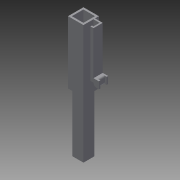
# Autodesk Inventor part: CraneArmLink1st
Saved by Autodesk Inventor 2015 (Build 190159000, 159)
## iProperties
Created: 2016-03-24
Part Number: CraneArmLink1st
Material: Generic
Document SubType Name: Modeling
Designer: Hatch
Density: 1 g/cm^3
Appearance: Default
Author: Hatch
Autodesk Inventor part; units mm, degrees
ref_plane "YZ Plane" through (0, 0, 0) normal (1, 0, 0) x (0, 1, 0)
ref_plane "XZ Plane" through (0, 0, 0) normal (0, 1, 0) x (-1, 0, 0)
ref_plane "XY Plane" through (0, 0, 0) normal (0, 0, 1) x (1, 0, 0)
sketch "Sketch1" plane through (0, 0, 0) normal (0, 1, 0) x (-1, 0, 0)
  line L0 (-7.125, 7.125) -> (7.125, 7.125)
  line L1 (7.125, 7.125) -> (7.125, -7.125)
  line L2 (7.125, -7.125) -> (-7.125, -7.125)
  line L3 (-7.125, -7.125) -> (-7.125, 7.125)
  line L4 (-7.125, 7.125) -> (7.125, -7.125) construction
  line L5 (7.125, 7.125) -> (-7.125, -7.125) construction
  point P0 (0, 0)
  dimension "d0" = 14.25
  dimension "d1" = 14.25
  constraints: 12 end point, 2 midpoint, 2 parallel, 1 horizontal, 1 perpendicular
  measures "d0" distance of L1.end L2.end
  measures "d1" distance of L0.end L1.end
extrude "Extrusion1" add sketch "Sketch1" along normal blind 76.2
sketch "Sketch2" plane through (0, 76.2, 0) normal (0, 1, 0) x (1, 0, 0)
  line L0 (10, -10) -> (-10, -10)
  line L1 (-10, -10) -> (-10, 10)
  line L2 (-10, 10) -> (10, 10)
  line L3 (10, 10) -> (10, -10)
  line L4 (10, -10) -> (-10, 10) construction
  line L5 (-10, -10) -> (10, 10) construction
  point P0 (0, 0)
  dimension "d4" = 20
  dimension "d5" = 20
  constraints: 12 end point, 2 midpoint, 2 parallel, 1 horizontal, 1 perpendicular
  measures "d4" distance of L1.end L2.end
  measures "d5" distance of L0.end L1.end
extrude "Extrusion2" add sketch "Sketch2" along normal blind 5
sketch "Sketch3" plane through (0, 81.2, 0) normal (0, 1, 0) x (1, 0, 0)
  line L0 (7.5, -7.5) -> (-7.5, -7.5)
  line L1 (-7.5, -7.5) -> (-7.5, 7.5)
  line L2 (-7.5, 7.5) -> (7.5, 7.5)
  line L3 (7.5, 7.5) -> (7.5, -7.5)
  line L4 (7.5, -7.5) -> (-7.5, 7.5) construction
  line L5 (-7.5, -7.5) -> (7.5, 7.5) construction
  line L6 (10, -10) -> (-10, -10)
  line L7 (-10, -10) -> (-10, 10)
  line L8 (-10, 10) -> (10, 10)
  line L9 (10, 10) -> (10, -10)
  line L10 (10, -10) -> (-10, 10) construction
  line L11 (-10, -10) -> (10, 10) construction
  point P0 (0, 0)
  dimension "d8" = 15
  dimension "d9" = 15
  constraints: 24 end point, 4 midpoint, 4 parallel, 2 horizontal, 2 perpendicular
  measures "d8" distance of L1.end L2.end
  measures "d9" distance of L0.end L1.end
extrude "Extrusion3" add sketch "Sketch3" along normal blind 76.2
sketch "Sketch4" plane through (10, 76.2, 10) normal (1, 0, 0) x (0, 0, -1)
  line L0 (20, 0) -> (20, 81.2) projected
  line L1 (15, 81.2) -> (15, 0)
  line L2 (0, 0) -> (20, 0) projected
  line L3 (15, 81.2) -> (13, 81.2)
  line L4 (17.5, 81.2) -> (2.5, 81.2) projected
  line L5 (13, 81.2) -> (13, 0)
  line L6 (13, 0) -> (15, 0)
  line L7 (20, 81.2) -> (0, 81.2) projected
  point P0 (10, -76.2)
  dimension "d12" = 2
  constraints: 8 end point, 3 point on line, 1 parallel, 1 perpendicular, 1 vertical
  measures "d12" distance of L1.start L3.end
extrude "Extrusion4" add sketch "Sketch4" along normal blind 10 contours L2 L5 L3 L1
sketch "Sketch5" plane through (10, 76.2, -3) normal (0, 0, 1) x (1, 0, 0)
  line L0 (0, 81.2) -> (10, 81.2) projected
  line L1 (10, 81.2) -> (8, 81.2)
  line L2 (8, 81.2) -> (8, 0)
  line L3 (8, 0) -> (10, 0)
  line L4 (10, 0) -> (10, 81.2)
  point P0 (-10, -76.2)
  dimension "d15" = 2
  constraints: 8 end point, 2 parallel, 1 perpendicular, 1 point on line
  measures "d15" distance of L0.end L1.end
extrude "Extrusion5" add sketch "Sketch5" along normal blind 8
sketch "Sketch6" plane through (20, 76.2, 10) normal (1, 0, 0) x (0, 0, -1)
  line L0 (5, 81.2) -> (3, 81.2)
  line L1 (3, 81.2) -> (3, 0)
  line L2 (3, 0) -> (5, 0)
  line L3 (5, 0) -> (5, 81.2)
  point P0 (10, -76.2)
  dimension "d18" = 2
  constraints: 8 end point, 2 parallel, 1 horizontal, 1 perpendicular
  measures "d18" distance of L0.start L0.end
extrude "Extrusion6" add sketch "Sketch6" against normal blind 4
sketch "Sketch7" plane through (10, 76.2, -5) normal (0, 0, -1) x (-1, 0, 0)
  line L0 (0, 0) -> (0, 81.2) projected
  line L1 (-10, 0) -> (0, 0)
  line L2 (0, 0) -> (0, 20)
  line L3 (0, 20) -> (-10, 20)
  line L4 (-10, 20) -> (-10, 0)
  point P0 (10, -76.2)
  dimension "d21" = 20
  constraints: 8 end point, 2 parallel, 1 horizontal, 1 perpendicular, 1 point on line
  measures "d21" distance of L2.end L1.end
extrude "Extrusion7" cut sketch "Sketch7" against normal through all
fillet "Fillet1" radius 5 1 edges at (18, 96.2, 1)
fillet "Fillet2" radius 2 1 edges at (18, 96.2, 5)
fillet "Fillet3" radius 2 1 edges at (15, 96.2, -3)
sketch "Sketch8" plane through (20, 76.2, 10) normal (1, 0, 0) x (0, 0, -1)
  line L0 (3, 81.2) -> (3, 20) projected
  line L1 (15, 20) -> (3, 20)
  line L2 (3, 20) -> (3, 25)
  line L3 (3, 25) -> (15, 25)
  line L4 (15, 25) -> (15, 20)
  line L5 (3, 20) -> (15, 20)
  line L6 (15, 20) -> (15, 16)
  line L7 (15, 16) -> (3, 16)
  line L8 (3, 16) -> (3, 20)
  point P0 (10, -76.2)
  dimension "d27" = 5
  dimension "d28" = 4
  constraints: 16 end point, 4 parallel, 2 horizontal, 2 perpendicular, 2 point on line
  measures "d27" distance of L1.end L2.end
  measures "d28" distance of L5.end L6.end
extrude "Extrusion8" add sketch "Sketch8" along normal blind 5
sketch "Sketch9" plane through (25, 76.2, 10) normal (1, 0, 0) x (0, 0, -1)
  line L0 (3, 16) -> (15, 16) projected
  line L1 (15, 25) -> (13, 25)
  line L2 (13, 25) -> (13, 16)
  line L3 (13, 16) -> (15, 16)
  line L4 (15, 16) -> (15, 25)
  line L5 (3, 25) -> (5, 25)
  line L6 (5, 25) -> (5, 16)
  line L7 (5, 16) -> (3, 16)
  line L8 (3, 16) -> (3, 25)
  point P0 (10, -76.2)
  dimension "d31" = 2
  dimension "d32" = 2
  constraints: 16 end point, 4 parallel, 2 horizontal, 2 perpendicular, 2 point on line
  measures "d31" distance of L3.end L2.end
  measures "d32" distance of L6.end L7.end
extrude "Extrusion9" add sketch "Sketch9" along normal blind 2
fillet "Fillet4" radius 2 1 edges at (25, 101.2, 1)
fillet "Fillet5" radius 2 1 edges at (25, 92.2, 1)
fillet "Fillet6" radius 4 1 edges at (20, 92.2, 1)
body "Solid1"
